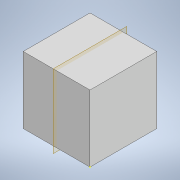
# Autodesk Inventor part: pawn
Saved by Autodesk Inventor 2021 (Build 250183000, 183)
## iProperties
Created: 2021-01-10
Part Number: pawn
Material: Generic
Document SubType Name: Modeling
Designer: Luke Kamols
Density: 1 g/cm^3
Appearance: Default
Author: Luke Kamols
Autodesk Inventor part; units mm, degrees
ref_plane "YZ Plane" through (0, 0, 0) normal (1, 0, 0) x (0, 1, 0)
ref_plane "XZ Plane" through (0, 0, 0) normal (0, 1, 0) x (-1, 0, 0)
ref_plane "XY Plane" through (0, 0, 0) normal (0, 0, 1) x (1, 0, 0)
sketch "Sketch1" plane through (0, 0, 0) normal (0, 1, 0) x (-1, 0, 0)
  point P0 (0, 0)
sketch "Sketch2" plane through (0, 0, 0) normal (0, 1, 0) x (-1, 0, 0)
  line L0 (0, 0) -> (16, 0)
  line L1 (16, 0) -> (16, -16)
  line L2 (16, -16) -> (0, -16)
  line L3 (0, -16) -> (0, 0)
  line L4 (0, 0) -> (0, -8)
  dimension "d1" = 16
  dimension "d2" = 16
  constraints: 10 end point, 2 parallel, 1 horizontal, 1 midpoint, 1 perpendicular
  measures "d1" distance of L1.end L2.end
  measures "d2" distance of L0.end L1.end
extrude "Extrusion1" add sketch "Sketch2" along normal blind 16
ref_plane "Work Plane1" through (-8, 0, 0) normal (1, 0, 0) x (0, 0, -1)
sketch "Sketch5" plane through (-8, 0, 0) normal (1, 0, 0) x (0, 0, -1)
  line L0 (0, 0) -> (16, 0) projected
  line L1 (11.3, 0) -> (4.7, 0) projected
  line L2 (8, 0) -> (11.3, 0)
  line L3 (11.3, 0) -> (11.3, 3.4)
  line L4 (11.3, 3.4) -> (10.9, 3.4)
  line L5 (11.3, 0) -> (11.3, 3.3) projected
  line L6 (10.9, 3.4) -> (11.3, 0)
  line L7 (11.3, 3.3) -> (8, 6.6) projected
  line L8 (8, 0) -> (8, 6.6)
  line L9 (10.9, 3.4) -> (8, 6.3)
  line L10 (16, 0) -> (0, 0)
  line L11 (5.1, 3.4) -> (4.7, 0)
  line L12 (5.1, 3.4) -> (8, 6.3)
  dimension "d39" = 3.3
  dimension "d40" = 3.4
  dimension "d41" = 0.4
  dimension "d42" = 6.6
  constraints: 18 end point, 3 symmetric about line, 2 perpendicular, 1 collinear, 1 midpoint, 1 point on line, 1 vertical
  measures "d39" distance of L2.start L1.start
  measures "d40" distance of L1.start L3.end
  measures "d41" distance of L3.end L4.end
  measures "d42" distance of L2.start L7.end
extrude "Extrusion4" cut sketch "Sketch5" along normal mid plane 13 contours L11 L12 L8 L0 | L8 L9 L6 L0
body "Solid1"
